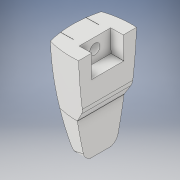
# Autodesk Inventor part: SCHUNK-1012603-FIN Co-act EGP 40/24
Saved by Autodesk Inventor 2019 (Build 230136000, 136)
## iProperties
Created: 2022-09-14
Part Number: SCHUNK-1012603-FIN Co-act EGP 40/24
Material: Generic
Catalog Web Link: www.cadenas.de
Description: FIN Co-act EGP-Finger Co-act EGP
Vendor: SCHUNK
Document SubType Name: Modeling
Designer: psAdmin
Manufacturer: SCHUNK
Mass: 14.606 g
Surface Area: 54.4272 cm^2
Volume: 14.606 cm^3
Density: 1 g/cm^3
Appearance: PSOLRGB-229-229-229
Category: PARTsolutions
Company: SCHUNK
Title: SCHUNK-1012603-FIN Co-act EGP 40/24
Author: Cadenas PARTsolutions
Comments: Finger Co-act EGP
PSOL_IDENT_0: {$CADENAS_DATA/23d-libs/schunk/greifsysteme/greifmodule/co_act/co_act_egp_c/fin_co_act_egp.prj},218
PSOL_IDENT_1: {VTYP=3D},{NB=SCHUNK-1012603-FIN Co-act EGP 40/24},{LINA=SCHUNK-1012603-FIN Co-act EGP 40/24},{NN=FI
PSOL_IDENT_2: N Co-act EGP},{DATE=21.12.2021 12:22:33},{GEOMDATE=21.11.2019 10:27:04},{VERSION=},{LINEID=20},{WBVA
PSOL_IDENT_3: R=},{WBNUMERIC=}  {NB=SCHUNK-1012603-FIN Co-act EGP 40/24},{LINA=SCHUNK-1012603-FIN Co-act EGP 40/24
PSOL_IDENT_4: },{KT=DUMMY},{IDNR=1012603},{TYP=FIN Co-act EGP 40/24},{TYP1=2.000},{R1=160.250},{L1=8.000},{A1=14.5
PSOL_IDENT_5: 00},{A2=0.000},{A3=0.000},{PARTSERVER=1},{B=0.000},{ANFGPKTEGH=0.000}
NB: SCHUNK-1012603-FIN Co-act EGP 40/24
NN: FIN Co-act EGP
NT: Finger Co-act EGP
NBSYN: SCHUNK-$IDNR.-$TYP.
LINA: SCHUNK-1012603-FIN Co-act EGP 40/24
CATALOG: SCHUNK
IDNR: 1012603
TYP: FIN Co-act EGP 40/24
TYP1: 2
R1: 160.25
L1: 8
A1: 14.5
A2: 0
A3: 0
PARTSERVER: 1
B: 0
ANFGPKTEGH: 0
SUPPLIER: SCHUNK
ARTICLENO: SCHUNK-1012603-FIN Co-act EGP 40/24
BOMINFO: SCHUNK-1012603-FIN Co-act EGP 40/24
CREATOR: CADENAS GmbH
Autodesk Inventor part; units mm, degrees
sketch "Sketch_1" plane through (0, 0, 0) normal (0, 0, 1) x (1, 0, 0)
  line L0 (0, 50) -> (0, 0)
  line L1 (0, 0) -> (20.15, 0)
  arc A0 (20.15, 0) -> (20.5, 0.35) centre (20.15, 0.35) ccw
  line L2 (20.5, 0.35) -> (20.5, 50)
  line L3 (20.5, 50) -> (0, 50)
  constraints: 8 end point, 2 point on circle, 1 centre point
extrude "Extrusion1" add sketch "Sketch_1" along normal mid plane 30
sketch "Sketch_23" plane through (0, 0, 0) normal (0, 0, 1) x (1, 0, 0)
  line L0 (14.5, 19.866) -> (14.5, 0)
  line L1 (14.5, 0) -> (20.5, 0)
  line L2 (20.5, 0) -> (20.5, 50)
  line L3 (20.5, 50) -> (18, 50)
  line L4 (18, 50) -> (18, 27.4019)
  arc A0 (17.3301, 24.9019) -> (18, 27.4019) centre (13, 27.4019) ccw
  line L5 (17.3301, 24.9019) -> (14.567, 20.116)
  arc A1 (14.567, 20.116) -> (14.5, 19.866) centre (15, 19.866) ccw
  constraints: 12 end point, 4 point on circle, 2 centre point
extrude "Extrusion2" cut sketch "Sketch_23" along normal mid plane 30
sketch "Sketch_4" plane through (0, 0, 0) normal (0, 0, 1) x (1, 0, 0)
  line L0 (49.5, 60) -> (49.5, -60)
  line L1 (-12, 50) -> (-12, 0)
  line L2 (-12, 0) -> (8, 0)
  arc A0 (0, 50) -> (8, 0) centre (160.25, 50) ccw
  line L3 (0, 50) -> (-12, 50)
  constraints: 8 end point, 2 point on circle, 1 centre point
revolve "Revolution1" cut sketch "Sketch_4" angle 55 mid plane about axis through (49.5, 60, 0) along (0, -1, 0)
sketch "Sketch_5" plane through (14.5, 0, 0) normal (1, 0, 0) x (0, 0, -1)
  line L0 (28, 60) -> (28, -60)
  line L1 (-28, 50) -> (-28, 0)
  line L2 (-28, 0) -> (-8, 0)
  arc A0 (-12, 20) -> (-8, 0) centre (284.0042, 68.8008) ccw
  arc A1 (-15, 50) -> (-12, 20) centre (221.5611, 58.5061) ccw
  line L3 (-15, 50) -> (-28, 50)
  constraints: 8 end point, 4 point on circle, 2 centre point
revolve "Revolution2" cut sketch "Sketch_5" angle 360 about axis through (14.5, 60, -28) along (0, 1, 0)
sketch "Sketch_6" plane through (14.5, 0, 0) normal (1, 0, 0) x (0, 0, -1)
  line L0 (-28, -60) -> (-28, 60)
  line L1 (8, 0) -> (28, 0)
  line L2 (28, 0) -> (28, 50)
  line L3 (28, 50) -> (15, 50)
  arc A0 (12, 20) -> (15, 50) centre (-221.5611, 58.5061) ccw
  arc A1 (8, 0) -> (12, 20) centre (-284.0042, 68.8008) ccw
  constraints: 8 end point, 4 point on circle, 2 centre point
revolve "Revolution3" cut sketch "Sketch_6" angle 360 about axis through (14.5, -60, 28) along (0, -1, 0)
sketch "Sketch_7" plane through (0, 0, 0) normal (0, 0, 1) x (1, 0, 0)
  line L0 (11.5, 38.4) -> (20.5, 38.4)
  line L1 (20.5, 38.4) -> (20.5, 50)
  line L2 (20.5, 50) -> (11.5, 50)
  line L3 (11.5, 50) -> (11.5, 38.4)
  constraints: 8 end point
extrude "Extrusion3" cut sketch "Sketch_7" along normal mid plane 16.2
sketch "Sketch_30" plane through (0, 0, 0) normal (1, 0, 0) x (0, 1, 0)
  line L0 (50, 6.5955) -> (6.4016, 4.1595)
  arc A0 (6.4016, 4.1595) -> (6.4016, -4.1595) centre (10, 0) ccw
  line L1 (6.4016, -4.1595) -> (50, -6.5955)
  line L2 (50, -6.5955) -> (50, -6.4925)
  line L3 (50, -6.4925) -> (6.4396, -4.06)
  arc A1 (6.4396, 4.06) -> (6.4396, -4.06) centre (10, 0) ccw
  line L4 (6.4396, 4.06) -> (50, 6.4925)
  line L5 (50, 6.4925) -> (50, 6.5955)
  constraints: 12 end point, 4 point on circle, 2 centre point
extrude "Extrusion4" cut sketch "Sketch_30" along normal blind 7
sketch "Sketch_31" plane through (0, 0, 0) normal (0, 0, 1) x (1, 0, 0)
  line L0 (20.5, 44.5) -> (0, 44.5)
  line L1 (0, 44.5) -> (0, 47.25)
  line L2 (0, 47.25) -> (2, 47.25)
  line L3 (2, 47.25) -> (2, 49)
  line L4 (2, 49) -> (7.75, 49)
  line L5 (7.75, 49) -> (7.75, 47.1)
  line L6 (7.75, 47.1) -> (20.5, 47.1)
  line L7 (20.5, 47.1) -> (20.5, 44.5)
  line L8 (20.5, 44.5) -> (0, 44.5)
  constraints: 18 end point
revolve "Revolution4" cut sketch "Sketch_31" angle 360 about axis through (20.5, 44.5, 0) along (1, 0, 0)
sketch "Sketch_13" plane through (0, 0, 0) normal (0, 0, 1) x (1, 0, 0)
  line L0 (0, 0.3578) -> (0, 0)
  line L1 (0, 0) -> (20.5, 0)
  line L2 (20.5, 0) -> (0, 0.3578)
  constraints: 6 end point
extrude "Extrusion5" cut sketch "Sketch_13" along normal mid plane 30
sketch "Sketch_26" plane through (0, 0, 0) normal (0, 0, 1) x (1, 0, 0)
  line L0 (49.5, 60) -> (49.5, -60)
  line L1 (-12, 50) -> (-12, 0)
  line L2 (-12, 0) -> (12.4087, 0)
  arc A0 (6.6579, 4.2885) -> (12.4087, 0) centre (12.4087, 6) ccw
  arc A1 (0, 50) -> (6.6579, 4.2885) centre (160.25, 50) ccw
  line L3 (0, 50) -> (-12, 50)
  constraints: 8 end point, 4 point on circle, 2 centre point
revolve "Revolution5" cut sketch "Sketch_26" angle 28 mid plane about axis through (49.5, 60, 0) along (0, -1, 0)
sketch "Sketch_28" plane through (18, 0, 0) normal (1, 0, 0) x (0, 0, -1)
  line L0 (8.1, 38.4) -> (8.3025, 38.4)
  line L1 (8.3025, 38.4) -> (8.1, 50)
  line L2 (8.1, 50) -> (8.1, 38.4)
  constraints: 6 end point
extrude "Extrusion6" cut sketch "Sketch_28" against normal blind 6.5
sketch "Sketch_27" plane through (18, 0, 0) normal (1, 0, 0) x (0, 0, -1)
  line L0 (-8.3025, 38.4) -> (-8.1, 38.4)
  line L1 (-8.1, 38.4) -> (-8.1, 50)
  line L2 (-8.1, 50) -> (-8.3025, 38.4)
  constraints: 6 end point
extrude "Extrusion7" cut sketch "Sketch_27" against normal blind 6.5
sketch "Sketch_29" plane through (0, 0, 0) normal (0, 0, 1) x (1, 0, 0)
  line L0 (11.5, 38.4) -> (18, 38.2865)
  line L1 (18, 38.2865) -> (18, 38.4)
  line L2 (18, 38.4) -> (11.5, 38.4)
  constraints: 6 end point
extrude "Extrusion8" cut sketch "Sketch_29" along normal mid plane 16.605
sketch "Sketch_19" plane through (0, 0, 0) normal (0, 0, 1) x (1, 0, 0)
  line L0 (0, 49.6858) -> (18, 50)
  line L1 (18, 50) -> (0, 50)
  line L2 (0, 50) -> (0, 49.6858)
  constraints: 6 end point
extrude "Extrusion9" cut sketch "Sketch_19" along normal mid plane 30
sketch "Sketch_9" plane through (14.5, 0, 0) normal (1, 0, 0) x (0, 0, -1)
  arc A0 (-8.8956, 3.9186) -> (-8, 0) centre (284.0042, 68.8008) ccw
  line L0 (-8, 0) -> (-4.014, 0)
  arc A1 (-8.8956, 3.9186) -> (-4.014, 0) centre (-4.014, 5) ccw
  constraints: 4 point on circle, 2 centre point, 2 end point
extrude "Extrusion10" cut sketch "Sketch_9" against normal blind 15
sketch "Sketch_11" plane through (14.5, 0, 0) normal (1, 0, 0) x (0, 0, -1)
  line L0 (4.014, 0) -> (8, 0)
  arc A0 (8, 0) -> (8.8956, 3.9186) centre (-284.0042, 68.8008) ccw
  arc A1 (4.014, 0) -> (8.8956, 3.9186) centre (4.014, 5) ccw
  constraints: 4 point on circle, 2 centre point, 2 end point
extrude "Extrusion11" cut sketch "Sketch_11" against normal blind 15
ref_plane "AUB_XY" through (14.5, 10, 0) normal (1, 0, 0) x (0, 0, -1)
ref_plane "AUB_YZ" through (14.5, 10, 0) normal (0, 0, -1) x (0, 1, 0)
ref_plane "AUB_ZX" through (14.5, 10, 0) normal (0, 1, 0) x (1, 0, 0)
ref_plane "AUB_DUMMY_XY" through (0, 0, 0) normal (0, 1, 0) x (1, 0, 0)
ref_plane "AUB_DUMMY_YZ" through (0, 0, 0) normal (1, 0, 0) x (0, 0, -1)
ref_plane "AUB_DUMMY_ZX" through (0, 0, 0) normal (0, 0, -1) x (0, 1, 0)
ref_plane "FIN_XY" through (11.5, 38.4, 0) normal (1, 0, 0) x (0, 0, -1)
ref_plane "FIN_YZ" through (11.5, 38.4, 0) normal (0, 0, -1) x (0, 1, 0)
ref_plane "FIN_ZX" through (11.5, 38.4, 0) normal (0, 1, 0) x (1, 0, 0)
body "Solid1"
